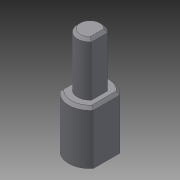
# Autodesk Inventor part: Shaft_Peg
Saved by Autodesk Inventor 2015 (Build 190159000, 159)
## iProperties
Created: 2014-08-17
Part Number: Shaft_Peg
Material: Generic
Document SubType Name: Modeling
Designer: User
Density: 1 g/cm^3
Appearance: Default
Author: User
Autodesk Inventor part; units mm, degrees
ref_plane "YZ Plane" through (0, 0, 0) normal (1, 0, 0) x (0, 1, 0)
ref_plane "XZ Plane" through (0, 0, 0) normal (0, 1, 0) x (-1, 0, 0)
ref_plane "XY Plane" through (0, 0, 0) normal (0, 0, 1) x (1, 0, 0)
sketch "Sketch1" plane through (0, 0, 0) normal (0, 0, 1) x (1, 0, 0)
  circle A0 centre (0, 0) radius 4
  line L0 (3.1225, 2.5) -> (3.1225, -2.5)
  line L1 (-3.1225, 2.5) -> (-3.1225, -2.5)
  dimension "d0" = 8
  dimension "d1" = 5
  dimension "d2" = 5
  constraints: 4 end point, 4 point on circle, 1 centre point, 1 coincident, 1 parallel, 1 vertical
  measures "d0" diameter of A0
  measures "d1" distance of L0.start L0.end
  measures "d2" distance of L1.start L1.end
extrude "Extrusion1" add sketch "Sketch1" along normal blind 10 contours L0 A0 L1
sketch "Sketch2" plane through (0, 0, 10) normal (0, 0, 1) x (1, 0, 0)
  circle A0 centre (0, 0) radius 2.35
  line L0 (1.809, 1.5) -> (1.809, -1.5)
  dimension "d5" = 4.7
  dimension "d6" = 3
  constraints: 2 end point, 2 point on circle, 1 centre point, 1 coincident, 1 vertical
  measures "d5" diameter of A0
  measures "d6" distance of L0.start L0.end
extrude "Extrusion2" add sketch "Sketch2" along normal blind 10 contours L0 A0 picked at (0.4227, 0)
chamfer "Chamfer1" distance 0.5 angle 45 6 edges at (1.809, 0, 20) (-2.35, 0, 20) (3.1225, 0, 10) (0, 4, 10) (0, -4, 10) (-3.1225, 0, 10)
body "Solid1"
